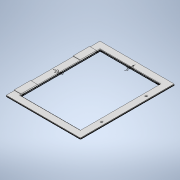
# Autodesk Inventor part: Tapa Superior
Saved by Autodesk Inventor 2022.6 (Build 266554000, 554)
## iProperties
Created: 2025-01-14
Part Number: Tapa Superior
Material: Genérico
Document SubType Name: Modeling
Designer: johan
Density: 1 g/cm^3
Appearance: Valor por defecto
Author: johan
Autodesk Inventor part; units mm, degrees
ref_plane "YZ Plane" through (0, 0, 0) normal (1, 0, 0) x (0, 1, 0)
ref_plane "XZ Plane" through (0, 0, 0) normal (0, 1, 0) x (-1, 0, 0)
ref_plane "XY Plane" through (0, 0, 0) normal (0, 0, 1) x (1, 0, 0)
sketch "Boceto1" plane through (0, 0, 0) normal (0, 1, 0) x (-1, 0, 0)
  line L0 (0, 0) -> (180, 0)
  line L1 (180, 0) -> (180, -240)
  line L2 (180, -240) -> (0, -240)
  line L3 (0, -240) -> (0, 0)
  line L4 (-3, -243) -> (183, -243)
  line L5 (183, -243) -> (183, 3)
  line L6 (183, 3) -> (-3, 3)
  line L7 (-3, 3) -> (-3, -243)
  line L8 (203, 23) -> (203, -263)
  line L9 (203, -263) -> (-23, -263)
  line L10 (-23, -263) -> (-23, 23)
  line L11 (-23, 23) -> (203, 23)
  dimension "d0" = 180
  dimension "d1" = 240
  dimension "d2" = 3
  dimension "d5" = 20
  constraints: 24 end point, 6 parallel, 3 perpendicular, 1 horizontal, 6 other
  measures "d0" distance of L1.end L2.end
  measures "d1" distance of L0.end L1.end
  measures "d2" distance between parallel lines of L2 L4
  measures "d5" distance between parallel lines of L5 L8
extrude "Extrusión3" add sketch "Boceto1" along normal blind 3 contours L8 L9 L10 L11
sketch "Boceto5" plane through (0, 3, 0) normal (0, 1, 0) x (1, 0, 0)
  line L0 (-203, 263) -> (-203, -23) projected
  line L1 (-183, -3) -> (-183, 243) projected
  line L2 (-203, 2) -> (-183, 2)
  line L3 (-183, 2) -> (-183, 52)
  line L4 (-183, 52) -> (-203, 52)
  line L5 (-203, 52) -> (-203, 2)
  line L6 (-203, 182) -> (-183, 182)
  line L7 (-183, 182) -> (-183, 232)
  line L8 (-183, 232) -> (-203, 232)
  line L9 (-203, 232) -> (-203, 182)
  line L10 (-203, -23) -> (23, -23) projected
  point P0 (0, 0)
  point P1 (-193, 182)
  dimension "d26" = 50
  dimension "d27" = 50
  dimension "d28" = 25
  dimension "d29" = 130
  constraints: 16 end point, 4 parallel, 4 point on line, 2 horizontal, 2 perpendicular, 1 midpoint
  measures "d26" distance of L3.end L2.end
  measures "d27" distance of L7.end L6.end
  measures "d28" distance between parallel lines of L10 L2
  measures "d29" distance from line of point (-193, 182) L4
extrude "Extrusión7" add sketch "Boceto5" along normal blind 1 contours L8 L1 L6 L0 | L4 L1 L2 L0
sketch "Boceto6" plane through (0, 3, 0) normal (0, 1, 0) x (1, 0, 0)
  line L0 (-203, 232) -> (-183, 232) projected
  line L1 (-183, 232) -> (-183, 243) projected
  line L2 (-183, 243) -> (3, 243) projected
  line L3 (3, 243) -> (3, -3) projected
  line L4 (3, -3) -> (-183, -3) projected
  line L5 (-183, -3) -> (-183, 2) projected
  line L6 (-183, 2) -> (-203, 2) projected
  line L7 (-203, 2) -> (-203, -23) projected
  line L8 (-203, -23) -> (23, -23) projected
  line L9 (23, -23) -> (23, 263) projected
  line L10 (23, 263) -> (-203, 263) projected
  line L11 (-203, 263) -> (-203, 232) projected
  line L12 (23, 91.3088) -> (23, 114.6899)
  line L13 (3, 114.6899) -> (3, 91.3088)
  circle A0 centre (13, 188) radius 3.175
  circle A1 centre (13, 52) radius 3.175
  point P0 (0, 0)
  dimension "d32" = 6.35
  dimension "d33" = 75
  dimension "d34" = 6.35
  dimension "d35" = 75
  constraints: 4 end point, 2 centre point, 2 point on line, 1 parallel
  measures "d32" diameter of A0
  measures "d33" distance from line of L10 A0.centre
  measures "d34" diameter of A1
  measures "d35" distance from line of L8 A1.centre
extrude "Extrusión8" cut sketch "Boceto6" against normal blind 3 contours A0 | A1
sketch "Boceto7" plane through (0, 4, 0) normal (0, 1, 0) x (1, 0, 0)
  line L0 (-203, 232) -> (-203, 182) projected
  line L1 (-203, 182) -> (-183, 182) projected
  line L2 (-183, 182) -> (-183, 232) projected
  line L3 (-183, 232) -> (-203, 232) projected
  line L4 (-203, 52) -> (-203, 2) projected
  line L5 (-203, 2) -> (-183, 2) projected
  line L6 (-183, 2) -> (-183, 52) projected
  line L7 (-183, 52) -> (-203, 52) projected
  line L8 (-203, 232) -> (-204, 232)
  line L9 (-204, 232) -> (-204, 182)
  line L10 (-204, 182) -> (-203, 182)
  line L11 (-203, 182) -> (-203, 232)
  line L12 (-203, 52) -> (-204, 52)
  line L13 (-204, 52) -> (-204, 2)
  line L14 (-204, 2) -> (-203, 2)
  line L15 (-203, 2) -> (-203, 52)
  point P0 (0, 0)
  dimension "d38" = 1
  dimension "d39" = 1
  constraints: 16 end point, 4 parallel, 2 horizontal, 2 perpendicular
  measures "d38" distance of L10.end L9.end
  measures "d39" distance of L14.end L13.end
extrude "Extrusión9" add sketch "Boceto7" against normal blind 5 contours L0 L10 L9 L8 | L4 L14 L13 L12
